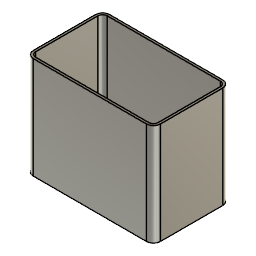
▢-125×75×2.3 (Autodesk Fusion 360 design; units mm, degrees)
Autodesk Fusion 360 part; units mm, degrees
sketch "スケッチ1" plane through (0, 0, 0) normal (0, 0, 1) x (1, 0, 0)
  line L0 (240.4841, -190.269) -> (351.6841, -190.269)
  line L1 (240.4841, -187.969) -> (351.6841, -187.969)
  line L2 (351.6841, -115.269) -> (240.4841, -115.269)
  line L3 (351.6841, -117.569) -> (240.4841, -117.569)
  arc A0 (233.5841, -183.369) -> (240.4841, -190.269) centre (240.4841, -183.369) ccw
  arc A1 (235.8841, -183.369) -> (240.4841, -187.969) centre (240.4841, -183.369) ccw
  arc A2 (240.4841, -115.269) -> (233.5841, -122.169) centre (240.4841, -122.169) ccw
  line L4 (233.5841, -122.169) -> (233.5841, -183.369)
  line L5 (235.8841, -122.169) -> (235.8841, -183.369)
  arc A3 (240.4841, -117.569) -> (235.8841, -122.169) centre (240.4841, -122.169) ccw
  arc A4 (351.6841, -190.269) -> (358.5841, -183.369) centre (351.6841, -183.369) ccw
  arc A5 (351.6841, -187.969) -> (356.2841, -183.369) centre (351.6841, -183.369) ccw
  line L6 (358.5841, -183.369) -> (358.5841, -122.169)
  line L7 (356.2841, -183.369) -> (356.2841, -122.169)
  arc A6 (358.5841, -122.169) -> (351.6841, -115.269) centre (351.6841, -122.169) ccw
  arc A7 (356.2841, -122.169) -> (351.6841, -117.569) centre (351.6841, -122.169) ccw
  point P0 (296.0841, -152.769)
extrude "押し出し1" add sketch "スケッチ1" along normal blind 100
